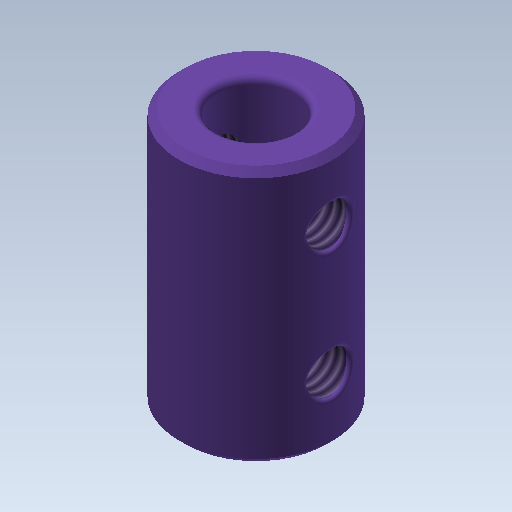
# Autodesk Inventor part: MOTOR COUPLER CONNECTOR
Saved by Autodesk Inventor 2021.1 (Build 251245010, 245A)
## iProperties
Created: 2022-09-23
Part Number: MOTOR COUPLER CONNECTOR
Material: Steel, Mild
Document SubType Name: Modeling
Designer: klama
Density: 7.85 g/cm^3
Appearance: Violet
Author: klama
Autodesk Inventor part; units mm, degrees
ref_plane "XZ Plane" through (0, 0, 0) normal (0, 1, 0) x (-1, 0, 0)
ref_plane "XY Plane" through (0, 0, 0) normal (0, 0, 1) x (1, 0, 0)
sketch "Sketch1" plane through (0, 0, 0) normal (0, 0, 1) x (1, 0, 0)
  line L0 (-1.2, 0) -> (7.2, 0) construction
  line L1 (0, -14) -> (0, 14) construction
  line L2 (3, 10) -> (3, -10)
  line L3 (3, -10) -> (6, -10)
  line L4 (6, -10) -> (6, 10)
  line L5 (6, 10) -> (3, 10)
  point P0 (0, 0)
  point P1 (3, 0)
  dimension "d0" = 12
  dimension "d1" = 6
  dimension "d2" = 20
  constraints: 8 end point, 3 perpendicular, 1 horizontal alignment, 1 midpoint, 1 vertical
  measures "d0" diameter of L4 L1
  measures "d1" diameter of L2 L1
  measures "d2" distance of L3.end L4.end
revolve "Revolution1" add sketch "Sketch1" angle 360 about axis through (0, -10, 0) along (0, 1, 0)
chamfer "Chamfer1" distance 0.5 angle 45 2 edges at (-6, 10, 0) (-6, -10, 0)
fillet "Fillet1" radius 0.5 2 edges at (-3, 10, 0) (-3, -10, 0)
sketch "Sketch2" plane through (0, 0, 0) normal (1, 0, 0) x (0, 1, 0)
  line L0 (-14, 0) -> (14, 0) construction
  line L1 (0, -8.4) -> (0, 8.4) construction
  line L2 (10, -3.5) -> (10, 3.5) projected
  point P0 (0, 0)
  point P1 (5, 0)
  dimension "d8" = 5
  constraints: 1 point on line
  measures "d8" distance from line of point (5, 0) L2
hole "Hole1" at (0, 5, 0) direction (-1, 0, 0) diameter 3.242 depth 11.8 tip angle 118 thread size "M4x0.7" class "6H" standard "ANSI Metric M Profile"
mirror "Mirror1" about plane through (0, 0, 0) normal (0, 1, 0) of "Hole1"
mirror "Mirror2" about plane through (0, 0, 0) normal (1, 0, 0) of "Hole1", "Mirror1"
fillet "Fillet2" radius 0.25 8 edges at (-5.7769, 4.9983, 1.621) (-5.7769, -4.9983, 1.621) (5.8744, 3.9339, -1.2211) (5.8746, 6.0668, -1.2205) (5.7769, 4.9998, 1.621) (5.8746, -6.0668, -1.2205) (5.8744, -3.9339, -1.2211) (5.7769, -4.9998, 1.621)
ref_plane "Work Plane2" through (6, 0, 0) normal (1, 0, 0) x (0, 1, 0)
ref_plane "Work Plane1" through (0, 0, 0) normal (1, 0, 0) x (0, 1, 0)
body "Solid1"
